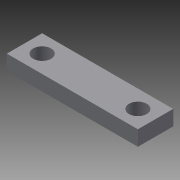
# Autodesk Inventor part: Transmitter clamp
Saved by Autodesk Inventor 2014 SP1 (Build 180222100, 222)
## iProperties
Created: 2014-05-13
Part Number: Transmitter clamp
Material: Generic
Document SubType Name: Modeling
Designer: Alex
Density: 1 g/cm^3
Appearance: Default
Author: Alex
Autodesk Inventor part; units mm, degrees
ref_plane "YZ Plane" through (0, 0, 0) normal (1, 0, 0) x (0, 1, 0)
ref_plane "XZ Plane" through (0, 0, 0) normal (0, 1, 0) x (-1, 0, 0)
ref_plane "XY Plane" through (0, 0, 0) normal (0, 0, 1) x (1, 0, 0)
sketch "Sketch1" plane through (0, 0, 0) normal (0, 0, 1) x (1, 0, 0)
  line L0 (0, 0) -> (26, 0)
  line L1 (26, 0) -> (26, 7)
  line L2 (26, 7) -> (0, 7)
  line L3 (0, 7) -> (0, 0)
  dimension "d0" = 26
  dimension "d1" = 7
  constraints: 8 end point, 2 parallel, 1 horizontal, 1 perpendicular
  measures "d0" distance of L2.end L1.end
  measures "d1" distance of L1.end L0.end
extrude "Extrusion1" add sketch "Sketch1" along normal blind 3
sketch "Sketch2" plane through (0, 0, 3) normal (0, 0, 1) x (1, 0, 0)
  line L0 (0, 0) -> (26, 0) projected
  line L1 (26, 7) -> (0, 7) projected
  line L2 (0, 7) -> (3.5739, 7)
  line L3 (3.5739, 0) -> (0, 0)
  line L4 (0, 0) -> (0, 7)
  line L5 (3.5739, 0) -> (22.546, 0)
  line L6 (22.546, 7) -> (3.5739, 7)
  line L7 (22.546, 7) -> (26, 7)
  line L8 (26, 7) -> (26, 0)
  line L9 (26, 0) -> (22.546, 0)
  line L10 (0, 0) -> (3.4896, 0)
  line L11 (3.4896, 7) -> (0, 7)
  line L12 (0, 7) -> (0, 0)
  line L13 (3.4896, 7) -> (22.4896, 7)
  line L14 (22.4896, 0) -> (3.4896, 0)
  line L15 (22.4896, 0) -> (26, 0)
  line L16 (26, 0) -> (26, 7)
  line L17 (26, 7) -> (22.4896, 7)
  line L18 (0, 0) -> (3.5, 0)
  line L19 (3.5, 0) -> (3.5, 7)
  line L20 (3.5, 7) -> (0, 7)
  line L21 (0, 7) -> (0, 0)
  line L22 (3.5, 0) -> (22.5, 0)
  line L23 (22.5, 0) -> (22.5, 7)
  line L24 (22.5, 7) -> (3.5, 7)
  line L25 (3.5, 7) -> (3.5, 0)
  line L26 (26, 0) -> (22.5, 0)
  line L27 (22.5, 0) -> (22.5, 3.5)
  line L28 (22.5, 3.5) -> (26, 3.5)
  line L29 (26, 3.5) -> (26, 0)
  circle A0 centre (3.5, 3.5) radius 1.7782
  circle A1 centre (22.5, 3.5) radius 1.7655
  dimension "d13" = 3.5
  dimension "d14" = 19
  dimension "d15" = 3.5564
  dimension "d16" = 3.531
  constraints: 56 end point, 12 parallel, 9 horizontal, 6 point on line, 5 perpendicular, 2 centre point, 2 midpoint, 1 coincident
  measures "d13" distance of L20.end L19.end
  measures "d14" distance of L24.end L23.end
  measures "d15" diameter of A0
  measures "d16" diameter of A1
extrude "Extrusion2" cut sketch "Sketch2" against normal blind 4.25 contours A0 L19 | L19 A0 | A1 L23 | L23 L28 A1 | L23 A1 L28
body "Solid1"
